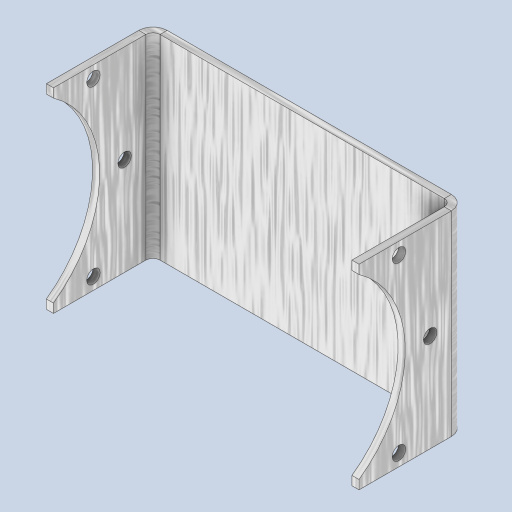
# Autodesk Inventor part: servo_arm
Saved by Autodesk Inventor 2023 (Build 270158000, 158)
## iProperties
Created: 2024-09-12
Part Number: servo_arm
Material: アルミニウム 5052
Document SubType Name: Sheet Metal
Designer: kiyo
Density: 2.68 g/cm^3
Sheet Metal Rule: アルミ5052_2mm
Appearance: サテン - ブラシ仕上げ 重厚
Author: kiyo
Autodesk Inventor part; units mm, degrees
ref_plane "YZ Plane" through (0, 0, 0) normal (1, 0, 0) x (0, 1, 0)
ref_plane "XZ Plane" through (0, 0, 0) normal (0, 1, 0) x (-1, 0, 0)
ref_plane "XY Plane" through (0, 0, 0) normal (0, 0, 1) x (1, 0, 0)
sketch "スケッチ2" plane through (0, 0, 0) normal (0, 0, 1) x (1, 0, 0)
  line L0 (44, -27.5) -> (-44, -27.5)
  line L1 (-44, -27.5) -> (-44, 27.5)
  line L2 (-44, 27.5) -> (44, 27.5)
  line L3 (44, 27.5) -> (44, -27.5)
  line L4 (44, -27.5) -> (-44, 27.5) construction
  line L5 (-44, -27.5) -> (44, 27.5) construction
  point P0 (0, 0)
  dimension "d5" = 88
  dimension "d6" = 55
  measures "d5" distance of L0.start L0.end
  measures "d6" distance of L0.end L1.end
extrude "プレート2" add sketch "スケッチ2" along normal blind 2
sketch "スケッチ3" plane through (42, 27.5, 0) normal (1, 0, 0) x (0, 1, 0)
  line L0 (-55, 0) -> (0, 0)
  line L1 (0, 0) -> (0, 30)
  line L2 (0, 30) -> (-55, 30)
  line L3 (-55, 30) -> (-55, 0)
  constraints: 6 end point, 1 horizontal, 1 perpendicular, 1 vertical
edge flange "フランジ1" height 30 angle 90 thickness 2 bend radius 2 thickness toward (1, 0, 0) relief tear relief width 2 relief depth 1 corner gap 2 corner form 0 edges at (44, 0, 2) (-44, 0, 2) wall of the first edge with corners at (42, -27.5, 0) (42, 27.5, 0) (42, 27.5, 30) (42, -27.5, 30)
bend "曲げ1"
corner "コーナー1"
sketch "スケッチ5" plane through (-44, -27.5, 30) normal (-1, 0, 0) x (0, 0, 1)
  circle A0 centre (17.5, 27.5) radius 37.5
  circle A1 centre (-11.2267, 3.3955) radius 1.8919
  circle A2 centre (10.9882, -9.4303) radius 1.8919
  circle A3 centre (36.25, -4.976) radius 1.8919
  circle A4 centre (52.7385, 14.6742) radius 1.8919
  circle A5 centre (52.7385, 40.3258) radius 1.8919
  circle A6 centre (36.25, 59.976) radius 1.8919
  circle A7 centre (10.9882, 64.4303) radius 1.8919
  circle A8 centre (-11.2267, 51.6045) radius 1.8919
  circle A9 centre (-20, 27.5) radius 1.8919
  line L0 (-26, 55) -> (-26, 0) projected
  circle A10 centre (17.5, 27.5) radius 30.5
  point P0 (-30, 27.5)
  dimension "d26" = 75
  dimension "d29" = 360
  dimension "d31" = 0
  dimension "d32" = 0
  dimension "d36" = 6
  dimension "d37" = 61
  constraints: 10 centre point, 1 coincident, 22 other
  measures "d31" vertical distance of point (-30, 27.5) point (17.5, 27.5)
  measures "d32" vertical distance of point (-30, 27.5) A9.centre
  measures "d36" distance from line of L0 A9.centre
  measures "d37" diameter of A10
extrude "押し出し1" cut sketch "スケッチ5" against normal up to surface (88 mm away) contours A8 A0 | A0 A8 | A1 A0 | A0 A1 | A9 A0 | A0 A9 | A10
equation "\"d7\" = Thickness"
equation "\"d8\" = BendReliefWidth"
equation "\"d9\" = BendReliefDepth"
equation "\"d10\" = MinimumRemnant"
equation "\"d11\" = TransitionRadius"
equation "\"d14\" = BendRadius"
equation "\"d15\" = CornerReliefSize"
equation "\"d16\" = GapSize"
equation "\"d17\" = JacobiRadiusSize"
equation "\"BendRadius\" = Thickness"
equation "\"BendReliefWidth\" = Thickness"
equation "\"BendReliefDepth\" = 0.5 * Thickness"
equation "\"CornerReliefSize\" = 4 * Thickness"
equation "\"MinimumRemnant\" = 2 * Thickness"
equation "\"TransitionRadius\" = BendRadius"
equation "\"JacobiRadiusSize\" = BendRadius"
equation "\"GapSize\" = Thickness"
equation "\"Thickness\" = 2"
